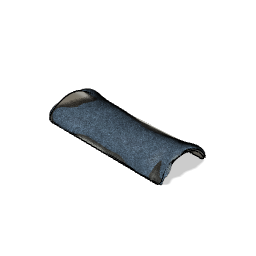
OpenHand (Autodesk Fusion 360 design; units mm, degrees)
Autodesk Fusion 360 part; units mm, degrees
other "Base Mesh Feature1"
sketch "Sketch1" plane through (0, 0, 0) normal (1, 0, 0) x (0, 0, -1)
  circle A0 centre (0, -14) radius 48
  circle A1 centre (0, -14) radius 51
  line L0 (0, 1.75) -> (0, 22.5)
  line L1 (41.9524, 15) -> (-41.9524, 15)
  dimension "d2" = 3
  dimension "d3" = 96
  dimension "d4" = 14
  dimension "d5" = 15
  constraint coincident A0.centre L0
  constraint coincident A1 L1.start
  constraint coincident A1 L1.end
  constraint horizontal L1
  measures "d3" diameter of A0
  measures "d4" distance of origin A0.centre
  measures "d5" distance of origin L1
ref_plane "WorkPlane1" through (220, 0, 0) normal (1, 0, 0) x (0, 1, 0)
sketch "Sketch2" plane through (220, 0, 0) normal (1, 0, 0) x (0, 0, -1)
  circle A0 centre (0, 4) radius 43
  line L0 (0, 1.75) -> (0, 22.5)
  circle A1 centre (0, 4) radius 46
  line L1 (-44.6654, 15) -> (44.6654, 15)
  dimension "d9" = 86
  dimension "d10" = 4
  dimension "d11" = 3
  dimension "d12" = 15
  constraint coincident A0.centre L0
  constraint coincident A1 L1.start
  constraint coincident A1 L1.end
  constraint horizontal L1
  measures "d9" diameter of A0
  measures "d10" distance of A0.centre origin
  measures "d12" distance of origin L1
loft "Loft1" add profiles "Sketch1", "Sketch2" section 1 contours A0 A1 L1 picked at (36.4034, 18.6695) section 2 contours A0 A1 L1 picked at (-42.9316, 17.1512) makes body 1
copy_body "Body->Comp1" bodies 1 removing the originals makes body 2 in component "Base"
ref_plane "WorkPlane2" through (0, 12.125, 0) normal (-0.906308, 0, -0.422618) x (0, 1, 0)
sketch "Sketch3" plane through (0, 0, 0) normal (-0.906308, 0, -0.422618) x (0, 1, 0)
  circle A0 centre (-5, 22) radius 30
  circle A1 centre (-5, 22) radius 33
  dimension "d16" = 60
  dimension "d17" = 5
  dimension "d18" = 22
  dimension "d19" = 3
  measures "d16" diameter of A0
  measures "d17" horizontal distance of origin A0.centre
  measures "d18" vertical distance of origin A0.centre
extrude "Extrude1" cut sketch "Sketch3" along normal mid plane 100 contours A0 | A1 bodies 2 in component "Base"
fillet "Fillet2" radius 8 5 edges at (0, 27.9469, -26.3393) (27.3545, 15, -40.4811) (220, 15, -43.1173) (220, 15, 43.1173) (0, 15, 40.1008) on bodies 2 in component "Base"
component "Base" placed x (1, 0, 0) y (0, 1, 0) z (0, 0, 1) at (0, 0, 0)
named bodies: "Base"
